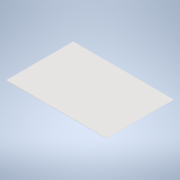
# Autodesk Inventor part: Part1
Saved by Autodesk Inventor 2022 (Build 260153000, 153)
## iProperties
Created: 2022-06-12
Part Number: Part1
Material: Generic
Document SubType Name: Modeling
Designer: logic
Density: 1 g/cm^3
Appearance: Default
Author: logic
Autodesk Inventor part; units mm, degrees
ref_plane "YZ Plane" through (0, 0, 0) normal (1, 0, 0) x (0, 1, 0)
ref_plane "XZ Plane" through (0, 0, 0) normal (0, 1, 0) x (-1, 0, 0)
ref_plane "XY Plane" through (0, 0, 0) normal (0, 0, 1) x (1, 0, 0)
sketch "Sketch1" plane through (0, 0, 0) normal (0, 1, 0) x (-1, 0, 0)
  line L0 (375, -250) -> (-375, -250)
  line L1 (-375, -250) -> (-375, 250)
  line L2 (-375, 250) -> (375, 250)
  line L3 (375, 250) -> (375, -250)
  point P0 (0, 0)
  dimension "d0" = 750
  dimension "d1" = 500
  dimension "d2" = 250
  dimension "d3" = 375
  constraints: 8 end point, 2 parallel, 1 horizontal, 1 perpendicular
  measures "d0" distance of L1.end L2.end
  measures "d1" distance of L0.end L1.end
  measures "d2" distance from line of point (0, 0) L0
  measures "d3" distance from line of L1 point (0, 0)
extrude "Extrusion1" add sketch "Sketch1" against normal blind 1
body "Solid1"
